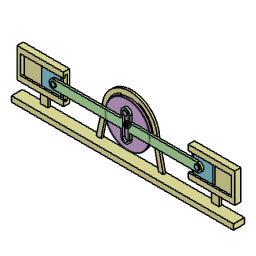
Scotch Yoke Mechanism v4 (Autodesk Fusion 360 design; units mm, degrees)
Autodesk Fusion 360 part; units mm, degrees
note: some values were not read from the file. Chosen so that the rebuilt part matches the saved one: which bodies a step acts on. Set by a fixed rule: which sketch regions a step uses.
sketch "crank" plane through (0, 0, 0) normal (0, 1, 0) x (1, 0, 0) in component "Crank"
  circle A0 centre (0, 0) radius 40
  dimension "d1" = 80
  constraint coincident A0.centre origin
  measures "d1" diameter of A0
extrude "Extrude1" add sketch "crank" along normal blind 4 makes body 1 in component "Crank"
sketch "Slider" plane through (0, 0, 0) normal (0, 1, 0) x (1, 0, 0) in component "Slider"
  line L0 (-190, 0) -> (-190, -20)
  line L1 (-155, -20) -> (-120, -20)
  line L2 (-120, -20) -> (-120, 0)
  line L3 (-120, 20) -> (-120, 0)
  line L4 (-155, 20) -> (-120, 20)
  line L5 (155, -20) -> (120, -20)
  line L6 (120, -20) -> (120, 0)
  line L7 (120, 20) -> (120, 0)
  line L8 (155, 20) -> (120, 20)
  line L9 (-155, -20) -> (-120, -20)
  line L10 (-120, -20) -> (-120, 20)
  line L11 (-120, 20) -> (-155, 20)
  line L12 (-155, 20) -> (-155, -20)
  line L13 (120, -20) -> (155, -20)
  line L14 (155, -20) -> (155, 20)
  line L15 (155, 20) -> (120, 20)
  line L16 (120, 20) -> (120, -20)
  dimension "d6" = 70
  dimension "d7" = 20
  dimension "d9" = 20
  constraint vertical L0
  constraint horizontal L1
  constraint vertical L2
  constraint horizontal L5
  constraint vertical L6
  constraint horizontal L9
  constraint vertical L10
  constraint horizontal L11
  constraint vertical L12
  constraint horizontal L13
  constraint vertical L14
  constraint horizontal L15
  constraint vertical L16
  measures "d6" distance of L2.end L0.start
  measures "d7" distance of L2.end L1.end
  measures "d9" distance of L6.end L5.end
extrude "Extrude1'" add sketch "Slider" along normal blind 4 separate body makes body 2 at (-143.3333, 0, -6.6667) makes body 3 at (143.3333, 0, 6.6667) in component "Slider"
sketch "holder" plane through (0, 0, 0) normal (0, 1, 0) x (1, 0, 0) in component "Holder"
  line L0 (-197, -27) -> (-113, -27)
  line L1 (-113, -27) -> (-113, 27)
  line L2 (-113, 27) -> (-197, 27)
  line L3 (-197, 27) -> (-197, -27)
  line L4 (197, 27) -> (113, 27)
  line L5 (113, 27) -> (113, -27)
  line L6 (113, -27) -> (197, -27)
  line L7 (197, -27) -> (197, 27)
  line L8 (0, 140) -> (0, 150)
  line L9 (230, 160) -> (-230, 160)
  line L10 (-230, 160) -> (-230, 140)
  line L11 (-230, 140) -> (230, 140)
  line L12 (230, 140) -> (230, 160)
  line L13 (230, 160) -> (-230, 140) construction
  line L14 (-230, 160) -> (230, 140) construction
  line L15 (50, 0) -> (80, 140)
  line L16 (-50, 0) -> (-80, 140)
  line L17 (-162, 27) -> (-148, 27)
  line L18 (-148, 27) -> (-148, 140)
  line L19 (-148, 140) -> (-162, 140)
  line L20 (-162, 140) -> (-162, 27)
  line L21 (148, 27) -> (162, 27)
  line L22 (162, 27) -> (162, 140)
  line L23 (162, 140) -> (148, 140)
  line L24 (148, 140) -> (148, 27)
  arc A0 (-50, 0) -> (50, 0) centre (0, 0) ccw
  point P0 (0, 150)
  dimension "d14" = 14
  dimension "d15" = 14
  dimension "d16" = 35
  dimension "d17" = 113
  dimension "d18" = 113
  dimension "d19" = 35
  constraint coincident A0.centre origin
  constraint vertical L8
  constraint horizontal L9
  constraint perpendicular L9 L10
  constraint parallel L9 L11
  constraint parallel L10 L12
  constraint coincident L13 P0
  constraint coincident L14 P0
  constraint coincident P0 L8.end
  constraint coincident L11 L15.end
  constraint symmetric L8 L15.start L16.start
  constraint symmetric L8 L15.end L16.end
  constraint horizontal L17
  constraint vertical L18
  constraint horizontal L19
  constraint vertical L20
  constraint coincident L2 L17.start
  constraint horizontal L21
  constraint vertical L22
  constraint horizontal L23
  constraint vertical L24
  constraint coincident L11 L22.end
  constraint coincident L4 L21.start
  constraint coincident L11 L8.start
  measures "d14" distance of L17.start L17.end
  measures "d15" distance of L21.start L21.end
  measures "d16" distance of L5 L24
  measures "d17" distance of A0.centre L5
  measures "d18" distance of L1 L8
  measures "d19" distance of L1 L18
extrude "Extrude1''" add sketch "holder" along normal blind 4 separate body contours L0 L1 L2 L3 L17 makes body 4 in component "Holder"
extrude "Extrude2" add sketch "holder" along normal blind 4 separate body contours L4 L5 L6 L7 L21 makes body 5 in component "Holder"
extrude "Extrude3" add sketch "holder" along normal blind 4 separate body contours L11 L15 L16 A0 makes body 6 in component "Holder"
extrude "Extrude4" add sketch "holder" along normal blind 4 contours L4 L11 L21 L22 L23 L24 bodies 5 in component "Holder"
extrude "Extrude5" add sketch "holder" along normal blind 4 contours L2 L11 L17 L18 L19 L20 bodies 4 in component "Holder"
extrude "Extrude6" add sketch "holder" along normal mid plane 20 contours L9 L10 L11 L12 L19 L23 bodies 4 5 6 in component "Holder"
move_body "Move1" bodies 2 to x (1, 0, 0) y (0, 1, 0) z (0, 0, 1) at (0, -25, 0) in component "Slider"
move_body "Move2" bodies 3 to x (1, 0, 0) y (0, 1, 0) z (0, 0, 1) at (0, -25, 0) in component "Slider"
sketch "left slider holder" plane through (0, 0, 0) normal (0, -1, 0) x (1, 0, 0) in component "Holder"
  line L0 (-197, 27) -> (-197, -27)
  line L1 (-197, -27) -> (-162, -27)
  line L2 (-162, -27) -> (-162, -140)
  line L3 (-162, -140) -> (-148, -140)
  line L4 (-148, -140) -> (-148, -27)
  line L5 (-148, -27) -> (-113, -27)
  line L6 (-113, -27) -> (-113, 27)
  line L7 (-113, 27) -> (-197, 27)
  line L8 (-197, 27) -> (-113, 27)
  line L9 (-113, 27) -> (-113, 21)
  line L10 (-113, 21) -> (-197, 21)
  line L11 (-197, 21) -> (-197, 27)
  line L12 (-197, -27) -> (-113, -27)
  line L13 (-113, -27) -> (-113, -21)
  line L14 (-113, -21) -> (-197, -21)
  line L15 (-197, -21) -> (-197, -27)
  line L16 (-197, 27) -> (-191, 27)
  line L17 (-191, 27) -> (-191, -27)
  line L18 (-191, -27) -> (-197, -27)
  line L19 (-197, -27) -> (-197, 27)
  dimension "d32" = 6
  dimension "d33" = 6
  dimension "d34" = 6
  dimension "d35" = 54
  constraint horizontal L8
  constraint vertical L9
  constraint horizontal L10
  constraint vertical L11
  constraint coincident L0.start L7.end
  constraint horizontal L12
  constraint vertical L13
  constraint horizontal L14
  constraint vertical L15
  constraint coincident L6 L13.end
  constraint coincident L0.end L1.start
  constraint horizontal L16
  constraint vertical L17
  constraint horizontal L18
  constraint vertical L19
  measures "d32" distance of L0.start L10.end
  measures "d33" distance of L0.end L14.end
  measures "d34" distance of L0.start L16.end
  measures "d35" distance of L0.start L0.end
extrude "Extrude7" add sketch "left slider holder" along normal blind 7 contours L0 L7 L8 L10 L11 L16 L17 L19 | L0 L10 L14 L17 L19 | L6 L7 L8 L9 L10 L17 | L0 L1 L12 L14 L15 L17 L18 L19 | L1 L5 L6 L12 L13 L14 L17 bodies 4 in component "Holder"
sketch "right slider holder" plane through (0, 0, 0) normal (0, -1, 0) x (1, 0, 0) in component "Holder"
  line L0 (113, 27) -> (113, -27)
  line L1 (113, -27) -> (148, -27)
  line L2 (148, -27) -> (148, -140)
  line L3 (148, -140) -> (162, -140)
  line L4 (162, -140) -> (162, -27)
  line L5 (162, -27) -> (197, -27)
  line L6 (197, -27) -> (197, 27)
  line L7 (197, 27) -> (113, 27)
  line L8 (113, 27) -> (197, 27)
  line L9 (197, 27) -> (197, 21)
  line L10 (197, 21) -> (113, 21)
  line L11 (113, 21) -> (113, 27)
  line L12 (113, -27) -> (197, -27)
  line L13 (197, -27) -> (197, -21)
  line L14 (197, -21) -> (113, -21)
  line L15 (113, -21) -> (113, -27)
  line L16 (197, 27) -> (191, 27)
  line L17 (191, 27) -> (191, -27)
  line L18 (191, -27) -> (197, -27)
  line L19 (197, -27) -> (197, 27)
  dimension "d38" = 6
  dimension "d39" = 6
  dimension "d40" = 6
  constraint horizontal L8
  constraint vertical L9
  constraint horizontal L10
  constraint vertical L11
  constraint coincident L0.start L7.end
  constraint horizontal L12
  constraint vertical L13
  constraint horizontal L14
  constraint vertical L15
  constraint coincident L6 L13.end
  constraint coincident L0.end L1.start
  constraint horizontal L16
  constraint vertical L17
  constraint horizontal L18
  constraint vertical L19
  constraint coincident L12 L17.end
  measures "d38" distance of L0.start L10.end
  measures "d39" distance of L0.end L14.end
  measures "d40" distance of L6.end L16.end
extrude "Extrude8" add sketch "right slider holder" along normal blind 7 contours L0 L7 L8 L10 L11 L17 | L6 L7 L8 L9 L10 L16 L17 L19 | L0 L1 L5 L12 L14 L15 L17 | L6 L10 L14 L17 L19 | L5 L6 L12 L13 L14 L17 L18 L19 bodies 4 in component "Holder"
sketch "left slider barrier top" plane through (0, 0, 21) normal (0, 0, -1) x (1, 0, 0) in component "Holder"
  line L0 (-191, 0) -> (-113, 0)
  line L1 (-113, 0) -> (-113, 7)
  line L2 (-113, 7) -> (-191, 7)
  line L3 (-191, 7) -> (-191, 0)
  line L4 (-113, 7) -> (-192, 7)
  line L5 (-192, 7) -> (-192, 4)
  line L6 (-192, 4) -> (-113, 4)
  line L7 (-113, 4) -> (-113, 7)
  dimension "d43" = 3
  constraint horizontal L4
  constraint vertical L5
  constraint horizontal L6
  constraint vertical L7
  constraint coincident L1.end L2.start
  measures "d43" distance of L1.end L6.end
sketch "left slider barrier bottom" plane through (0, 0, -21) normal (0, 0, 1) x (-1, 0, 0) in component "Holder"
  line L0 (113, 0) -> (191, 0)
  line L1 (191, 0) -> (191, 7)
  line L2 (191, 7) -> (113, 7)
  line L3 (113, 7) -> (113, 0)
  line L4 (191, 7) -> (113, 7)
  line L5 (113, 7) -> (113, 4)
  line L6 (113, 4) -> (191, 4)
  line L7 (191, 4) -> (191, 7)
  dimension "d44" = 3
  constraint horizontal L4
  constraint vertical L5
  constraint horizontal L6
  constraint vertical L7
  constraint coincident L1.end L2.start
  measures "d44" distance of L1.end L6.end
extrude "Extrude9" add sketch "left slider barrier top" along normal blind 4 contours L1 L2 L3 L4 L6 L7 bodies 4 in component "Holder"
extrude "Extrude10" add sketch "left slider barrier bottom" along normal blind 4 contours L1 L2 L3 L4 L5 L6 L7 bodies 4 in component "Holder"
sketch "right slider barrier top" plane through (0, 0, 21) normal (0, 0, -1) x (1, 0, 0) in component "Holder"
  line L0 (113, 0) -> (191, 0)
  line L1 (191, 0) -> (191, 7)
  line L2 (191, 7) -> (113, 7)
  line L3 (113, 7) -> (113, 0)
  line L4 (113, 7) -> (191, 7)
  line L5 (191, 7) -> (191, 4)
  line L6 (191, 4) -> (113, 4)
  line L7 (113, 4) -> (113, 7)
  dimension "d49" = 3
  constraint horizontal L4
  constraint vertical L5
  constraint horizontal L6
  constraint vertical L7
  constraint coincident L1 L5.end
  constraint coincident L2.end L3.start
  measures "d49" distance of L2.end L6.end
sketch "right slider barrier bottom" plane through (0, 0, -21) normal (0, 0, 1) x (-1, 0, 0) in component "Holder"
  line L0 (-191, 0) -> (-113, 0)
  line L1 (-113, 0) -> (-113, 7)
  line L2 (-113, 7) -> (-191, 7)
  line L3 (-191, 7) -> (-191, 0)
  line L4 (-113, 7) -> (-191, 7)
  line L5 (-191, 7) -> (-191, 4)
  line L6 (-191, 4) -> (-113, 4)
  line L7 (-113, 4) -> (-113, 7)
  dimension "d50" = 3
  constraint horizontal L4
  constraint vertical L5
  constraint horizontal L6
  constraint vertical L7
  constraint coincident L1.end L2.start
  constraint coincident L2.end L3.start
  measures "d50" distance of L1.end L6.end
extrude "Extrude11" add sketch "right slider barrier bottom" along normal blind 4 contours L1 L2 L3 L4 L5 L6 L7 bodies 4 in component "Holder"
extrude "Extrude12" add sketch "right slider barrier top" along normal blind 4 contours L1 L2 L3 L4 L5 L6 L7 bodies 4 in component "Holder"
sketch "Sketch2" plane through (0, 0, 0) normal (0, -1, 0) x (1, 0, 0) in component "Crank"
  circle A0 centre (0, 0) radius 40
  circle A1 centre (0, 0) radius 5
  dimension "d55" = 10
  constraint concentric A0 A1
  measures "d55" diameter of A1
extrude "Extrude2'" cut sketch "Sketch2" against normal blind 45 contours A1 bodies 1 in component "Crank"
extrude "Extrude13" add sketch "Sketch2" along normal blind -6 and the other way blind -1 contours A1 sketch seen with x (1, 0, 0) y (0, 1, 0) z (0, 0, 1) at (0, -4, 0) bodies 4 in component "Holder"
move_face "OffsetFaces1" offset -0.3 1 faces at (4.9752, -3.3333, -0.4978) on bodies 4 in component "Holder"
sketch "Sketch1" plane through (-0.493, 20.9215, 0.3555) normal (0, 1, 0) x (-1, 0, 0) in component "Connecting rod"
sketch "Connection rod" plane through (0, -4, 0) normal (0, 1, 0) x (1, 0, 0) in component "Connecting rod"
  line L0 (-120, 0) -> (-130, 0)
  line L1 (120, 0) -> (130, 0)
  circle A0 centre (-130, 0) radius 5
  circle A1 centre (130, 0) radius 5
  line L2 (0, 0) -> (0, 20)
  line L3 (7.9965, 7.9728) -> (8, 19.9977)
  line L4 (-130.3859, -7.9907) -> (-7.9918, -7.9549)
  line L5 (-130.3859, 7.9907) -> (-129.6188, 7.9909)
  line L6 (-7.9965, 7.9909) -> (-130.3859, 7.9907)
  line L7 (7.9942, -7.9728) -> (129.9982, -8)
  line L8 (129.9982, 8) -> (7.9965, 7.9728)
  line L9 (-5, -20) -> (-5, 20)
  line L10 (5, -20) -> (5, 20)
  arc A2 (-7.9884, -19.5701) -> (7.9884, -19.5701) centre (0, -20) ccw
  arc A3 (-5, -20) -> (5, -20) centre (0, -20) ccw
  arc A4 (8, 19.9977) -> (-8, 19.9977) centre (0, 20) ccw
  arc A5 (5, 20) -> (-5, 20) centre (0, 20) ccw
  arc A6 (-129.6141, 7.9907) -> (-129.6094, -7.9905) centre (-130, 0) ccw
  arc A7 (129.9982, -8) -> (122, 0) centre (130, 0) ccw
  line L11 (-7.9884, -19.5701) -> (-7.9918, -7.9549)
  line L12 (-7.9965, 7.9909) -> (-8, 19.9977)
  line L13 (7.9884, -19.5701) -> (7.9942, -7.9728)
  dimension "d63" = 10
  dimension "d64" = 10
  dimension "d65" = 10
  dimension "d66" = 10
  constraint horizontal L0
  constraint horizontal L1
  constraint coincident L0.end A0.centre
  constraint coincident L1.end A1.centre
  constraint coincident L2.start origin
  constraint coincident L2.end A4.centre
  constraint tangent L3 A4
  constraint tangent A4 L11
  constraint coincident L4.start A6
  constraint perpendicular L4 L11
  constraint coincident L5.start A6
  constraint coincident L5.end A6
  constraint perpendicular L5 L11
  constraint coincident L6.start L11
  constraint tangent L7 A7
  constraint coincident L8.start A7
  constraint tangent L8 A7
  constraint tangent L9 A5
  constraint parallel L2 L9
  constraint tangent L10 A5
  constraint vertical L10
  constraint concentric A2 A3
  constraint concentric A4 A5
  constraint concentric A0 A6
  constraint coincident L4 A6.end
  constraint coincident L6 A6.start
  constraint concentric A1 A7
  constraint coincident L1 A7.end
  constraint collinear L11 L12
  measures "d63" diameter of A3
  measures "d64" diameter of A0
  measures "d65" diameter of A1
  measures "d66" diameter of A5
extrude "Extrude1'''" add sketch "Connection rod" against normal blind 4 separate body contours L3 L4 L5 L6 L7 L8 A2 A4 A6 A7 L11 L12 L13 makes body 7 in component "Connecting rod"
sketch "conection point" plane through (0, 0, 0) normal (0, -1, 0) x (1, 0, 0) in component "Crank"
  circle A0 centre (0, 20) radius 4
  dimension "d73" = 8
  measures "d73" diameter of A0
extrude "Extrude3'" add sketch "conection point" along normal blind -5 and the other way blind -5 bodies 1 in component "Crank"
sketch "Sketch2 (2)" plane through (0, -25, 0) normal (0, -1, 0) x (1, 0, 0) in component "Slider"
  line L0 (-155, 20) -> (-155, -20)
  line L1 (-155, -20) -> (-120, -20)
  line L2 (-120, -20) -> (-120, 20)
  line L3 (-120, 20) -> (-155, 20)
  circle A0 centre (-129.5, 0) radius 4
  dimension "d78" = 8
  measures "d78" diameter of A0
extrude "Extrude2''" add sketch "Sketch2 (2)" along normal blind -2 and the other way blind -5 contours A0 bodies 2 in component "Slider"
sketch "Sketch3" plane through (0, -25, 0) normal (0, -1, 0) x (1, 0, 0) in component "Slider"
  line L0 (120, 20) -> (120, -20)
  line L1 (120, -20) -> (155, -20)
  line L2 (155, -20) -> (155, 20)
  line L3 (155, 20) -> (120, 20)
  circle A0 centre (130.5, 0) radius 4
  dimension "d83" = 8
  measures "d83" diameter of A0
extrude "Extrude3''" add sketch "Sketch3" along normal blind -3.5 and the other way blind -5 contours A0 bodies 3 in component "Slider"
sketch "Sketch8" plane through (0, 0, 0) normal (0, -1, 0) x (1, 0, 0) in component "Holder"
  line L0 (-50, 0) -> (-80, -140)
  line L1 (-80, -140) -> (80, -140)
  line L2 (80, -140) -> (50, 0)
  arc A0 (50, 0) -> (-50, 0) centre (0, 0) ccw
  line L3 (42.4054, -1.3352) -> (70, -140)
  line L4 (-42.4054, -1.3352) -> (-70, -140)
  spline S0 degree 5 poles (-15.7017, 39.4139) (-15.1096, 35.3521) (-13.9224, 27.5835) (-12.1321, 16.9952) (-9.7258, 5.0423) (-6.6838, -6.0463) (-3.6046, -12.9387) (-0.4851, -15.2936) (2.6762, -12.9265) (5.8777, -6.0266) (9.1164, 5.0631) (11.7346, 17.0112) (13.7126, 27.5927) (15.0376, 35.3554) (15.7017, 39.4139) knots 0 0 0 0 0 0 0.1 0.2 0.3 0.4 0.5 0.6 0.7 0.8 0.9 1 1 1 1 1 1
  arc A1 (42.4054, -1.3352) -> (-42.4054, -1.3352) centre (0, 0) ccw
  circle A2 centre (0, 0) radius 4.7
  point P0 (-0.4939, -14.1161)
  constraint coincident A0.centre A1.centre
  constraint coincident L1 L3.end
  constraint coincident L1 L4.end
  constraint coincident S0.start A1
  constraint coincident S0.end A1
extrude "Extrude14" cut sketch "Sketch8" against normal blind 40 contours L1 L3 L4 S0 A1 bodies 4 in component "Holder"
sketch "Sketch1 (2)" plane through (0, 0, 0) normal (0, 1, 0) x (1, 0, 0)
  line L0 (-250, 50) -> (300, 50)
  line L1 (300, 50) -> (300, 250)
  line L2 (300, 250) -> (-250, 250)
  line L3 (-250, 250) -> (-250, 50)
  constraint horizontal L0
  constraint perpendicular L0 L1
  constraint perpendicular L1 L2
  constraint perpendicular L2 L3
extrude "Extrude15" cut sketch "Sketch1 (2)" along normal mid plane 240 bodies 4 makes body 8 at (4.1007, 4, 18.6712) makes body 9 at (157.3333, 4, 9) in component "Holder"
sketch "Sketch2 (3)" plane through (0, 0, 0) normal (0, 0, 1) x (1, 0, 0)
sketch "bottom" plane through (0, 0, 0) normal (0, 0, 1) x (1, 0, 0) in component "Holder"
  line L0 (-200.2117, 5.9422) -> (201.7255, 5.9422)
  line L1 (201.7255, 5.9422) -> (201.7255, -13.9065)
  line L2 (201.7255, -13.9065) -> (-200.2117, -13.9065)
  line L3 (-200.2117, -13.9065) -> (-200.2117, 5.9422)
  constraint horizontal L0
  constraint vertical L1
  constraint horizontal L2
  constraint vertical L3
extrude "Extrude16" add sketch "bottom" against normal blind 10 separate body makes body 10 in component "Holder"
move_body "Move1'" bodies 10 to x (1, 0, 0) y (0, 1, 0) z (0, 0, 1) at (0, 0, -50) in component "Holder"
combine "Combine1" operation add target body 8 tool bodies 10 4 9 in component "Holder"
component "Crank" placed x (1, 0, 0) y (0, 1, 0) z (0, 0, 1) at (0, -4, 0)
component "Slider" placed x (1, 0, 0) y (0, 1, 0) z (0, 0, 1) at (-0.493, 20.9215, 0.3555)
component "Holder" placed x (1, 0, 0) y (0, 1, 0) z (0, 0, 1) at (0, 0, 0)
component "Connecting rod" placed x (1, 0, 0) y (0, 1, 0) z (0, 0, 1) at (0, 0, 0)
named bodies: "Crank", "Slider Left", "Slider Right", "Holder", "Holder (1)", "Holder (2)"
